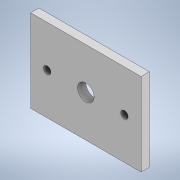
# Autodesk Inventor part: Soporte Piston
Saved by Autodesk Inventor 2021 (Build 250183000, 183)
## iProperties
Created: 2021-05-02
Part Number: Soporte Piston
Material: Generic
Document SubType Name: Modeling
Designer: maaro
Density: 1 g/cm^3
Appearance: Default
Author: maaro
Autodesk Inventor part; units mm, degrees
ref_plane "YZ Plane" through (0, 0, 0) normal (1, 0, 0) x (0, 1, 0)
ref_plane "XZ Plane" through (0, 0, 0) normal (0, 1, 0) x (-1, 0, 0)
ref_plane "XY Plane" through (0, 0, 0) normal (0, 0, 1) x (1, 0, 0)
sketch "Sketch2" plane through (0, 0, 0) normal (0, 0, 1) x (1, 0, 0)
  line L0 (0, 0) -> (200, 0)
  line L1 (200, 0) -> (200, 150)
  line L2 (200, 150) -> (0, 150)
  line L3 (0, 150) -> (0, 0)
  circle A0 centre (100, 75) radius 15
  dimension "d4" = 150
  dimension "d5" = 200
  dimension "d6" = 75
  dimension "d7" = 100
  dimension "d8" = 30
  constraints: 8 end point, 2 parallel, 1 centre point, 1 horizontal, 1 perpendicular
  measures "d4" distance of L2.end L0.start
  measures "d5" distance of L1.end L2.end
  measures "d6" distance from line of A0.centre L2
  measures "d7" distance from line of A0.centre L3
  measures "d8" diameter of A0
extrude "Extrusion2" add sketch "Sketch2" against normal blind 15
sketch "Sketch3" plane through (0, 0, 0) normal (0, 0, 1) x (1, 0, 0)
  line L0 (200, 150) -> (0, 150) projected
  line L1 (0, 150) -> (0, 0) projected
  point P0 (30, 75)
  point P1 (170, 75)
  dimension "d11" = 75
  dimension "d12" = 75
  dimension "d13" = 140
  dimension "d14" = 30
  measures "d11" distance from line of point (30, 75) L0
  measures "d12" distance from line of point (170, 75) L0
  measures "d13" distance of point (170, 75) point (30, 75)
  measures "d14" distance from line of point (30, 75) L1
hole "Hole1" at (30, 75, 0) at (170, 75, 0) direction (0, 0, -1) diameter 13.3858 end through all thread size "5/8-11 UNC" class "2B" standard "ANSI Unified Screw Threads"
thread "Thread1" size "M30x1.5" class "6H" standard "ANSI Metric M Profile" length 25
equation "\"d12\" = d11"
body "Solid2"
